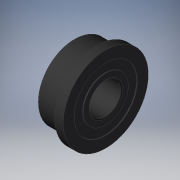
# Autodesk Inventor part: C-EFL683ZZ
Saved by Autodesk Inventor 2019 (Build 230136000, 136)
## iProperties
Created: 2024-09-02
Part Number: C-EFL683ZZ
Material: Generic
Catalog Web Link: www.cadenas.de
Description: C-EFL6__ZZ-Economy Miniature Deep Groove Ball Bearing - Double Shielded, Flanged
Vendor: MISUMI
Document SubType Name: Modeling
Designer: psAdmin
Manufacturer: MISUMI
Mass: 0.101849 g
Surface Area: 1.95228 cm^2
Volume: 0.101849 cm^3
Density: 1 g/cm^3
Appearance: PSOLRGB-175-175-175
Category: PARTsolutions
Company: MISUMI
Title: C-EFL683ZZ
Author: Cadenas PARTsolutions
Comments: Economy Miniature Deep Groove Ball Bearing - Double Shielded, Flanged
PSOL_IDENT_0: {$CADENAS_DATA/23d-libs/misumi/metric/12_bearing_holders/c_efl673zz.prj},165 {VTYP=3D},{NB=C-EFL683Z
PSOL_IDENT_1: Z},{LINA=C-EFL683ZZ},{NN=C-EFL6__ZZ},{DATE=29.05.2023 02:13:13},{GEOMDATE=25.05.2021 01:25:46},{VERS
PSOL_IDENT_2: ION=},{LINEID=230},{WBVAR=},{WBNUMERIC=}  {NB=C-EFL683ZZ},{LINA=C-EFL683ZZ},{KT=DUMMY},{PN=C-EFL683Z
PSOL_IDENT_3: Z},{TS=C-EFL683ZZ},{DD=3},{D=7},{B=3.0},{D1=8.1},{C=0.8},{RR=0.10},{R=0.10},{AA=2.8400},{BB=0.4970},
PSOL_IDENT_4: {C1=0.6400}
NB: C-EFL683ZZ
NN: C-EFL6__ZZ
NT: Economy Miniature Deep Groove Ball Bearing - Double Shielded, Flanged
NBSYN: $PN.
LINA: C-EFL683ZZ
CATALOG: Misumi
PN: C-EFL683ZZ
TS: C-EFL683ZZ
DD: 3
D: 7
B: 3
D1: 8.1
C: 0.8
RR: 0.1
SUPPLIER: MISUMI
ARTICLENO: C-EFL683ZZ
BOMINFO: C-EFL683ZZ
CREATOR: CADENAS GmbH
Autodesk Inventor part; units mm, degrees
ref_plane "YZ Plane" through (0, 0, 0) normal (1, 0, 0) x (0, 1, 0)
ref_plane "XZ Plane" through (0, 0, 0) normal (0, 1, 0) x (-1, 0, 0)
ref_plane "XY Plane" through (0, 0, 0) normal (0, 0, 1) x (1, 0, 0)
sketch "Sketch_1" plane through (0, 0, 0) normal (0, 0, 1) x (1, 0, 0)
  line L0 (7, 0) -> (-7, 0)
  arc A0 (0, 1.6) -> (0.1, 1.5) centre (0.1, 1.6) ccw
  line L1 (0.1, 1.5) -> (2.9, 1.5)
  arc A1 (2.9, 1.5) -> (3, 1.6) centre (2.9, 1.6) ccw
  line L2 (3, 1.6) -> (3, 2.14)
  line L3 (3, 2.14) -> (2.92, 2.14)
  line L4 (2.92, 2.14) -> (2.92, 3.003)
  line L5 (2.92, 3.003) -> (3, 3.003)
  line L6 (3, 3.003) -> (3, 4.05)
  line L7 (3, 4.05) -> (2.2, 4.05)
  line L8 (2.2, 4.05) -> (2.2, 3.6)
  arc A2 (2.1, 3.5) -> (2.2, 3.6) centre (2.2, 3.5) ccw
  line L9 (2.1, 3.5) -> (0.1, 3.5)
  arc A3 (0.1, 3.5) -> (0, 3.4) centre (0.1, 3.4) ccw
  line L10 (0, 3.4) -> (0, 3.003)
  line L11 (0, 3.003) -> (0.08, 3.003)
  line L12 (0.08, 3.003) -> (0.08, 2.14)
  line L13 (0.08, 2.14) -> (0, 2.14)
  line L14 (0, 2.14) -> (0, 1.6)
  constraints: 30 end point, 8 point on circle, 4 centre point
revolve "Revolution1" add sketch "Sketch_1" angle 360 about axis through (7, 0, 0) along (1, 0, 0)
ref_plane "to_housing_XY" through (0, 0, 0) normal (1, 0, 0) x (0, 0, -1)
ref_plane "to_housing_YZ" through (0, 0, 0) normal (0, 0, -1) x (0, 1, 0)
ref_plane "to_housing_ZX" through (0, 0, 0) normal (0, 1, 0) x (1, 0, 0)
body "Solid1"
